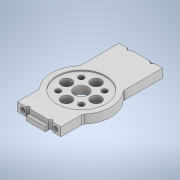
# Autodesk Inventor part: Leg_joint_yaw_frame
Saved by Autodesk Inventor 2020.4 (Build 244396000, 396)
## iProperties
Created: 2021-09-21
Part Number: Leg_joint_yaw_frame
Material: アルミニウム 2014-T4
Document SubType Name: Modeling
Designer: Masato Kubotera
Density: 2.8 g/cm^3
Appearance: 滑らか - 淡い灰色
Description: A2017 T5
Author: Masato Kubotera
Autodesk Inventor part; units mm, degrees
ref_plane "YZ Plane" through (0, 0, 0) normal (1, 0, 0) x (0, 1, 0)
ref_plane "XZ Plane" through (0, 0, 0) normal (0, 1, 0) x (-1, 0, 0)
ref_plane "XY Plane" through (0, 0, 0) normal (0, 0, 1) x (1, 0, 0)
sketch "スケッチ1" plane through (0, 0, 0) normal (0, 0, 1) x (1, 0, 0)
  line L0 (-12.5, 29.25) -> (12.5, 29.25)
  line L1 (12.5, 29.25) -> (12.5, -29.25)
  line L2 (12.5, -29.25) -> (-12.5, -29.25)
  line L3 (-12.5, -29.25) -> (-12.5, 29.25)
  line L4 (-12.5, 29.25) -> (12.5, -29.25) construction
  line L5 (12.5, 29.25) -> (-12.5, -29.25) construction
  line L6 (-5.5, 29.25) -> (-5.5, 31.25)
  line L7 (-5.5, 31.25) -> (5.5, 31.25)
  line L8 (0, 29.25) -> (0, -29.25) construction
  line L9 (5.5, 29.25) -> (5.5, 31.25)
  arc A0 (-7.6, 29.25) -> (-5.5, 29.25) centre (-6.55, 29.25) ccw
  arc A1 (5.5, 29.25) -> (7.6, 29.25) centre (6.55, 29.25) ccw
  line L10 (-12.5, 0) -> (12.5, 0) construction
  line L11 (-5.5, -29.25) -> (-5.5, -31.25)
  line L12 (-5.5, -31.25) -> (5.5, -31.25)
  line L13 (5.5, -29.25) -> (5.5, -31.25)
  arc A2 (-5.5, -29.25) -> (-7.6, -29.25) centre (-6.55, -29.25) ccw
  arc A3 (7.6, -29.25) -> (5.5, -29.25) centre (6.55, -29.25) ccw
  circle A4 centre (0, -5) radius 13.95 construction
  circle A5 centre (0, -5) radius 14.05
  circle A6 centre (-6.6998, -11.6998) radius 1.55
  line L14 (-9.9349, -14.9349) -> (0, -5) construction
  circle A7 centre (6.6998, -11.6998) radius 1.55
  circle A8 centre (6.6998, 1.6998) radius 1.55
  circle A9 centre (-6.6998, 1.6998) radius 1.55
  circle A10 centre (0, -5) radius 4
  circle A11 centre (0, -13.5) radius 3
  circle A12 centre (8.5, -5) radius 3
  circle A13 centre (0, 3.5) radius 3
  circle A14 centre (-8.5, -5) radius 3
  arc A15 (-10.6051, 8.3504) -> (-12.5, -16.5954) centre (0, -5) ccw
  arc A16 (12.5, -16.5954) -> (10.6051, 8.3504) centre (0, -5) ccw
  point P0 (0, 0)
  point P1 (-5.5, -29.25)
  point P2 (5.5, -29.25)
  point P3 (7.6, 29.25)
  point P4 (5.5, -29.25)
  point P5 (-5.5, -29.25)
  point P6 (-12.5, 1.415)
  point P7 (12.5, 1.415)
  point P8 (12.5, -11.415)
  point P9 (-12.5, -11.415)
  point P10 (12.5, -16.5954)
  point P11 (12.5, 6.5954)
  point P12 (-12.5, 6.5954)
  dimension "d0" = 25
  dimension "d1" = 58.5
  dimension "d2" = 11
  dimension "d3" = 2
  dimension "d4" = 1.05
  dimension "d13" = 27.9
  dimension "d17" = 24.25
  dimension "d44" = 0.1
  dimension "d48" = 3.1
  dimension "d49" = 45
  dimension "d50" = 9.475
  dimension "d53" = 360
  dimension "d55" = 8
  dimension "d56" = 6
  dimension "d57" = 8.5
  dimension "d60" = 360
  dimension "d64" = 3
  constraints: 30 end point, 16 centre point, 14 symmetric about line, 12 point on circle, 7 point on line, 6 midpoint, 4 coincident, 3 perpendicular, 2 parallel, 1 horizontal, 25 other
  measures "d0" distance of L1.end L2.end
  measures "d1" distance of L0.end L1.end
  measures "d2" distance of L7.end L6.end
  measures "d3" vertical distance of L0.end L7.end
  measures "d4" radius of A0
  measures "d13" diameter of A4
  measures "d17" distance of L8.end A4.centre
  measures "d48" diameter of A6
  measures "d49" angle of L8 L14
  measures "d50" distance of A6.centre point (0, -5)
  measures "d55" diameter of A10
  measures "d56" diameter of A11
  measures "d57" distance of point (0, -5) A11.centre
extrude "押し出し1" add sketch "スケッチ1" along normal blind 5 contours L0 A0 A1 L1 A5 L3 | L3 A5 A15 | L3 A5 L1 L2 A3 A2 | L1 A16 A5
extrude "押し出し2" add sketch "スケッチ1" along normal blind 2.5 contours L6 L7 L9 L0 | L2 L13 L12 L11
sketch "スケッチ2" plane through (-12.5, -29.25, 0) normal (0, -1, 0) x (1, 0, 0)
  line L0 (0, 0) -> (4.9, 0) projected
  line L1 (12.5, 5) -> (12.5, 0) construction
  line L2 (0, 0) -> (25, 0) projected
  line L3 (0, 5) -> (25, 5) projected
  point P0 (3, 2.5)
  point P1 (22, 2.5)
  point P2 (20.1, 0)
  point P3 (7, 5)
  point P4 (18, 5)
  point P5 (7, 0)
  dimension "d26" = 2.5
  dimension "d27" = 19
  constraints: 2 end point, 1 midpoint, 1 symmetric about line, 1 vertical
  measures "d26" distance from line of L0 point (3, 2.5)
  measures "d27" distance of point (22, 2.5) point (3, 2.5)
hole "穴1" at (-9.5, -29.25, 2.5) at (9.5, -29.25, 2.5) direction (0, 1, 0) diameter 2.459 depth 8 tip angle 118 thread size "M3x0.5" class "6H" standard "ISO Metric profile"
sketch "スケッチ3" plane through (-12.5, 29.25, 0) normal (0, 1, 0) x (1, 0, 0)
  circle A0 centre (22, -2.5) radius 1.2295 projected
  circle A1 centre (3, -2.5) radius 1.2295 projected
  point P0 (12.5, 0)
  constraints: 2 coincident
hole "穴2" at (9.5, 29.25, 2.5) at (-9.5, 29.25, 2.5) direction (0, -1, 0) diameter 2.459 depth 8 tip angle 118 thread size "M3x0.5" class "6H" standard "ISO Metric profile"
extrude "押し出し3" add sketch "スケッチ1" along normal blind 4.5 contours A5 L1 L3 | L3 A5 | A5 L1
fillet "フィレット3" radius 2 4 edges at (-12.5, -16.5954, 2.5) (-12.5, 6.5954, 2.5) (12.5, 6.5954, 2.5) (12.5, -16.5954, 2.5)
